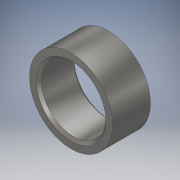
# Autodesk Inventor part: Axel Buffer
Saved by Autodesk Inventor 2018 (Build 220112000, 112)
## iProperties
Created: 2018-02-28
Part Number: Axel Buffer
Material: Stainless Steel
Document SubType Name: Modeling
Designer: 232963
Density: 8 g/cm^3
Appearance: Semi-Polished
Author: 232963
Autodesk Inventor part; units mm, degrees
ref_plane "YZ Plane" through (0, 0, 0) normal (1, 0, 0) x (0, 1, 0)
ref_plane "XZ Plane" through (0, 0, 0) normal (0, 1, 0) x (-1, 0, 0)
ref_plane "XY Plane" through (0, 0, 0) normal (0, 0, 1) x (1, 0, 0)
sketch "Sketch1" plane through (0, 0, 0) normal (0, 0, 1) x (1, 0, 0)
  circle A0 centre (0, 0) radius 4.0704
  circle A1 centre (0, 0) radius 5.2388
  dimension "d0" = 8.1407
  dimension "d1" = 1.1684
  constraints: 2 centre point, 2 coincident
  measures "d0" diameter of A0
  measures "d1" radial gap between concentric circles of A0 A1
extrude "Extrusion1" add sketch "Sketch1" along normal blind 4.7625
chamfer "Chamfer1" distance 0.3175 angle 45 2 edges at (-4.0704, 0, 4.7625) (-4.0704, 0, 0)
body "Solid1"
